# Autodesk Inventor part: DS3234
Saved by Autodesk Inventor 2016 (Build 200138000, 138)
## iProperties
Created: 2016-04-08
Part Number: DS3234
Material: Generic
Document SubType Name: Modeling
Designer: Paschalis
Density: 1 g/cm^3
Appearance: DS3234, DS3234
Author: Paschalis
Autodesk Inventor part; units mm, degrees
ref_plane "YZ Plane" through (0, 0, 0) normal (1, 0, 0) x (0, 1, 0)
ref_plane "XZ Plane" through (0, 0, 0) normal (0, 1, 0) x (-1, 0, 0)
ref_plane "XY Plane" through (0, 0, 0) normal (0, 0, 1) x (1, 0, 0)
sketch "DS3234, DS3234_61" plane through (0, 0, 0) normal (0, 0, 1) x (1, 0, 0)
  line L0 (-6.5, 3.877) -> (6.627, 3.877)
  line L1 (6.627, 3.877) -> (6.627, -3.877)
  line L2 (6.627, -3.877) -> (-6.5, -3.877)
  line L3 (-6.5, -3.877) -> (-6.5, 3.877)
  constraints: 8 end point
extrude "Extrusion1" add sketch "DS3234, DS3234_61" along normal blind 1
body "Solid1"
